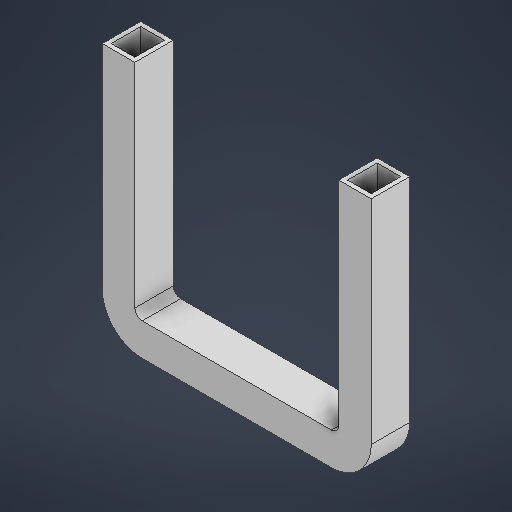
# Autodesk Inventor part: Part3
Saved by Autodesk Inventor 2026 (Build 300175050, 175E)
## iProperties
Created: 2026-04-23
Part Number: Part3
Material: Generic
Document SubType Name: Modeling
Designer: Administrator
Density: 1 g/cm^3
Appearance: Default
Author: Administrator
Autodesk Inventor part; units mm, degrees
ref_plane "YZ Plane" through (0, 0, 0) normal (1, 0, 0) x (0, 1, 0)
ref_plane "XZ Plane" through (0, 0, 0) normal (0, 1, 0) x (-1, 0, 0)
ref_plane "XY Plane" through (0, 0, 0) normal (0, 0, 1) x (1, 0, 0)
sketch "Sketch3" plane through (0, 0, 0) normal (0, 0, 1) x (1, 0, 0)
  line L0 (0, 0) -> (0, -72)
  line L1 (8, -80) -> (72, -80)
  line L2 (80, -72) -> (80, 0)
  arc A0 (0, -72) -> (8, -80) centre (8, -72) ccw
  arc A1 (72, -80) -> (80, -72) centre (72, -72) ccw
  point P0 (0, -80)
  point P1 (80, -80)
  dimension "d0" = 80
  dimension "d1" = 80
  dimension "d2" = 8
  constraints: 6 end point, 4 point on circle, 4 point on line, 4 tangent, 2 centre point, 2 perpendicular, 1 equal radius, 1 vertical
  measures "d0" distance of L0.start point (0, -80)
  measures "d1" distance of point (0, -80) point (80, -80)
  measures "d2" radius of A0
sketch "Sketch4" plane through (0, 0, 0) normal (0, 1, 0) x (-1, 0, 0)
  line L0 (4, -5) -> (-4, -5)
  line L1 (-4, -5) -> (-4, 5)
  line L2 (-4, 5) -> (4, 5)
  line L3 (4, 5) -> (4, -5)
  line L4 (4, -5) -> (-4, 5) construction
  line L5 (-4, -5) -> (4, 5) construction
  line L6 (5.5, -6.5) -> (-5.5, -6.5)
  line L7 (-5.5, -6.5) -> (-5.5, 6.5)
  line L8 (-5.5, 6.5) -> (5.5, 6.5)
  line L9 (5.5, 6.5) -> (5.5, -6.5)
  point P0 (0, 0)
  dimension "d3" = 8
  dimension "d4" = 10
  dimension "d5" = 1.5
  constraints: 20 end point, 4 parallel, 2 midpoint, 2 perpendicular, 1 horizontal, 3 other
  measures "d3" distance of L1.end L2.end
  measures "d4" distance of L0.end L1.end
  measures "d5" distance between parallel lines of L3 L9
sweep "Sweep1" add profiles "Sketch4" path "Sketch3"
body "Solid1"
